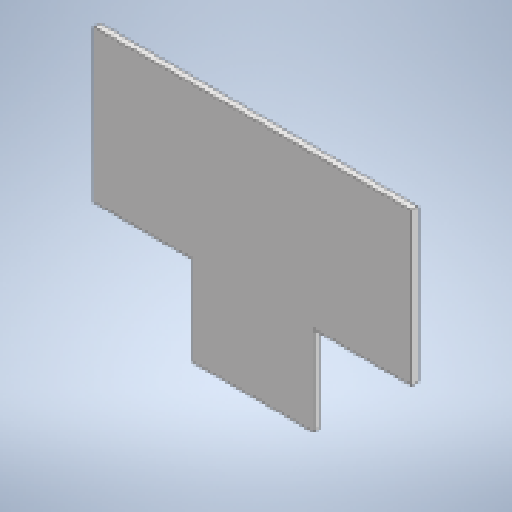
# Autodesk Inventor part: pokrywa
Saved by Autodesk Inventor 2023 (Build 270158000, 158)
## iProperties
Created: 2025-01-11
Part Number: pokrywa
Material: Ogólny
Document SubType Name: Modeling
Designer: kamil
Density: 1 g/cm^3
Appearance: Domyślna
Author: kamil
Autodesk Inventor part; units mm, degrees
ref_plane "YZ Plane" through (0, 0, 0) normal (1, 0, 0) x (0, 1, 0)
ref_plane "XZ Plane" through (0, 0, 0) normal (0, 1, 0) x (-1, 0, 0)
ref_plane "XY Plane" through (0, 0, 0) normal (0, 0, 1) x (1, 0, 0)
sketch "Szkic1" plane through (0, 0, 0) normal (0, 0, 1) x (1, 0, 0)
  line L0 (54, -20) -> (54, -3) projected
  line L1 (16, -31) -> (54, -31) projected
  circle A0 centre (35, -25.5) radius 3.5 projected
  circle A1 centre (26, -7) radius 3.5 projected
  circle A2 centre (44, -7) radius 3.5 projected
  line L2 (16, -31) -> (54, -31) projected
  line L3 (54, -20) -> (54, -31) projected
  line L4 (54, -20) -> (54, -3) projected
  line L5 (54, -3) -> (16, -3) projected
  line L6 (16, -3) -> (16, -20) projected
  line L7 (16, -31) -> (16, -20) projected
  line L8 (85, -3) -> (85, 41.8489) projected
  line L9 (-15, 44.8489) -> (85, 44.8489) projected
  line L10 (-15, -3) -> (-15, 41.8489) projected
  line L11 (-15, -4) -> (15.8, -4)
  line L12 (85, 44.8489) -> (-15, 44.8489)
  line L13 (-15, 44.8489) -> (-15, -3)
  line L14 (-15, -3) -> (85, -3)
  line L15 (85, -3) -> (85, 44.8489)
  line L16 (54, -31) -> (16, -31)
  line L17 (16, -31) -> (16, -3)
  line L18 (16, -3) -> (54, -3)
  line L19 (54, -3) -> (54, -31)
  point P0 (0, 0)
  constraints: 18 end point, 4 parallel, 3 horizontal, 2 perpendicular, 2 other
extrude "Wyciągnięcie proste1" add sketch "Szkic1" along normal blind 2 contours L3 L1 L7 L6 L5 L0 | L5 L14 L10 L13 L9 L15 L8 | A0 | A1 | A2
